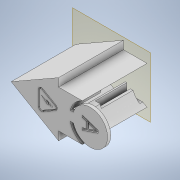
# Autodesk Inventor part: Wire_Closing_3
Saved by Autodesk Inventor 2022.3 (Build 263350000, 350)
## iProperties
Created: 2023-05-07
Part Number: Wire_Closing_3
Material: Generic
Document SubType Name: Modeling
Designer: Manuel Hueso Béjar
Density: 1 g/cm^3
Appearance: Default
Author: Manuel Hueso Béjar
Autodesk Inventor part; units mm, degrees
ref_plane "YZ Plane" through (0, 0, 0) normal (1, 0, 0) x (0, 1, 0)
ref_plane "XZ Plane" through (0, 0, 0) normal (0, 1, 0) x (-1, 0, 0)
ref_plane "XY Plane" through (0, 0, 0) normal (0, 0, 1) x (1, 0, 0)
ref_plane "Work Plane1" through (0, 0, 0) normal (0, 0, 1) x (1, 0, 0)
sketch "Sketch1" plane through (0, 0, 0) normal (0, 0, 1) x (1, 0, 0)
  line L0 (7.4997, 17.3208) -> (7.4997, 12.145) projected
  line L1 (-22.5003, 0.1452) -> (7.4997, 17.3208) projected
  line L2 (7.4997, -17.3208) -> (-22.5003, 0.1452) projected
  line L3 (7.4997, -11.855) -> (7.4997, -17.3208) projected
  line L4 (22.5003, -11.855) -> (7.4997, -11.855) projected
  arc A0 (19.8352, -10.355) -> (22.5003, -11.855) centre (27.4997, 0.1452) ccw projected
  line L5 (5.9997, -10.355) -> (19.8352, -10.355) projected
  line L6 (5.9997, -14.7118) -> (5.9997, -10.355) projected
  line L7 (-19.5003, 0.1343) -> (5.9997, -14.7118) projected
  line L8 (5.9997, 14.7336) -> (-19.5003, 0.1343) projected
  line L9 (5.9997, 10.645) -> (5.9997, 14.7336) projected
  line L10 (19.8345, 10.645) -> (5.9997, 10.645) projected
  arc A1 (22.4991, 12.145) -> (19.8345, 10.645) centre (27.4997, 0.1452) ccw projected
  line L11 (7.4997, 12.145) -> (22.4991, 12.145) projected
  point P0 (0, 0)
extrude "Extrusion1" add sketch "Sketch1" along normal blind 41
sketch "Sketch2" plane through (0, 0, 41) normal (0, 0, 1) x (1, 0, 0)
  line L0 (-22.5003, 0.1452) -> (7.4997, -17.3208) projected
  line L1 (7.4997, -17.3208) -> (7.4997, -11.855) projected
  line L2 (7.4997, -11.855) -> (22.5003, -11.855) projected
  arc A0 (19.8352, -10.355) -> (22.5003, -11.855) centre (27.4997, 0.1452) ccw projected
  line L3 (19.8352, -10.355) -> (5.9997, -10.355) projected
  line L4 (5.9997, -10.355) -> (5.9997, -14.7118) projected
  line L5 (5.9997, -14.7118) -> (-19.5003, 0.1343) projected
  line L6 (-19.5003, 0.1343) -> (5.9997, 14.7336) projected
  line L7 (5.9997, 14.7336) -> (5.9997, 10.645) projected
  line L8 (5.9997, 10.645) -> (19.8345, 10.645) projected
  arc A1 (22.4991, 12.145) -> (19.8345, 10.645) centre (27.4997, 0.1452) ccw projected
  line L9 (22.4991, 12.145) -> (7.4997, 12.145) projected
  line L10 (7.4997, 12.145) -> (7.4997, 17.3208) projected
  line L11 (7.4997, 17.3208) -> (-22.5003, 0.1452) projected
  arc A2 (22.4991, 12.145) -> (19.8345, 10.645) centre (27.4997, 0.1452) ccw projected
  arc A3 (22.4991, 12.145) -> (22.5003, -11.855) centre (27.4997, 0.1452) ccw
  arc A4 (16.9167, -2.8548) -> (16.9167, 3.1452) centre (27.4997, 0.1452) ccw projected
  line L12 (16.9167, -2.8548) -> (14.8506, -2.8548) projected
  arc A5 (14.8506, -2.8548) -> (14.8506, 3.1452) centre (27.4997, 0.1452) ccw projected
  line L13 (14.8506, 3.1452) -> (16.9167, 3.1452) projected
  point P0 (0, 0)
  constraints: 3 point on circle, 2 end point, 1 centre point, 1 coincident
extrude "Extrusion2" add sketch "Sketch2" against normal blind 2 contours L3 L4 L5 L6 L7 L8 A3 | A3 L13 A4 L12
sketch "Sketch3" plane through (0, 0, 39) normal (0, 0, -1) x (-1, 0, 0)
  line L0 (-15.4997, 5.1452) -> (-13.8506, 5.1452) projected
  line L1 (-13.8506, 5.1452) -> (-11.8506, 7.1452) projected
  line L2 (-11.8506, 7.1452) -> (-11.8506, 3.1452) projected
  line L3 (-11.8506, 3.1452) -> (-14.8506, 3.1452) projected
  arc A0 (-14.8506, 3.1452) -> (-15.4997, 5.1452) centre (-27.4997, 0.1452) ccw projected
  arc A1 (-15.4997, -4.8548) -> (-14.8506, -2.8548) centre (-27.4997, 0.1452) ccw projected
  line L4 (-14.8506, -2.8548) -> (-11.8506, -2.8548) projected
  line L5 (-11.8506, -2.8548) -> (-11.8506, -6.8548) projected
  line L6 (-11.8506, -6.8548) -> (-13.8506, -4.8548) projected
  line L7 (-13.8506, -4.8548) -> (-15.4997, -4.8548) projected
  line L8 (-5.9997, 14.7336) -> (19.5003, 0.1343) projected
  line L9 (-5.9997, 10.645) -> (-5.9997, 14.7336) projected
  line L10 (-19.8345, 10.645) -> (-5.9997, 10.645) projected
  arc A2 (-14.8506, 3.1452) -> (-19.8345, 10.645) centre (-27.4997, 0.1452) ccw projected
  line L11 (-14.8506, 3.1452) -> (-16.9167, 3.1452) projected
  arc A3 (-16.9167, 3.1452) -> (-16.9167, -2.8548) centre (-27.4997, 0.1452) ccw projected
  line L12 (-16.9167, -2.8548) -> (-14.8506, -2.8548) projected
  arc A4 (-19.8352, -10.355) -> (-14.8506, -2.8548) centre (-27.4997, 0.1452) ccw projected
  line L13 (-5.9997, -10.355) -> (-19.8352, -10.355) projected
  line L14 (-5.9997, -14.7118) -> (-5.9997, -10.355) projected
  line L15 (19.5003, 0.1343) -> (-5.9997, -14.7118) projected
  line L16 (-13.9334, -5.0548) -> (-11.6506, -7.3376)
  line L17 (-11.6506, -7.3376) -> (-11.6506, -2.6548)
  line L18 (-11.6506, -2.6548) -> (-15.0097, -2.6548)
  arc A5 (-15.8035, -5.0548) -> (-15.0097, -2.6548) centre (-27.4997, 0.1452) ccw
  line L19 (-15.8035, -5.0548) -> (-13.9334, -5.0548)
  line L20 (-11.6506, 2.9452) -> (-11.6506, 7.6281)
  line L21 (-11.6506, 7.6281) -> (-13.9334, 5.3452)
  line L22 (-13.9334, 5.3452) -> (-15.8035, 5.3452)
  arc A6 (-15.0097, 2.9452) -> (-15.8035, 5.3452) centre (-27.4997, 0.1452) ccw
  line L23 (-15.0097, 2.9452) -> (-11.6506, 2.9452)
  line L24 (-11.8506, -2.8548) -> (-11.6506, -2.8548)
  line L25 (-11.8506, 3.1452) -> (-11.6506, 3.1452)
  line L26 (-10.6506, -9.7518) -> (-14.3476, -6.0548)
  line L27 (-14.3476, -6.0548) -> (-17.4598, -6.0548)
  arc A7 (-17.4598, -6.0548) -> (-15.8378, -1.6548) centre (-27.4997, 0.1452) ccw
  line L28 (-15.8378, -1.6548) -> (-10.6506, -1.6548)
  line L29 (-10.6506, -1.6548) -> (-10.6506, -9.7518)
  line L30 (-14.3476, 6.3452) -> (-10.6506, 10.0423)
  line L31 (-10.6506, 10.0423) -> (-10.6506, 1.9452)
  line L32 (-10.6506, 1.9452) -> (-15.8378, 1.9452)
  arc A8 (-15.8378, 1.9452) -> (-17.4598, 6.3452) centre (-27.4997, 0.1452) ccw
  line L33 (-17.4598, 6.3452) -> (-14.3476, 6.3452)
  line L34 (-11.6506, -2.8548) -> (-10.6506, -2.8548)
  line L35 (-11.6506, 3.1452) -> (-10.6506, 3.1452)
  point P0 (0, 0)
  point P1 (-16.0734, 6.3452)
  point P2 (-15.585, 5.3452)
  point P3 (-15.585, -5.0548)
  point P4 (-16.0734, -6.0548)
  dimension "d4" = 0.2
  dimension "d5" = 0.2
  dimension "d6" = 1
  dimension "d7" = 1
  constraints: 40 end point, 8 point on circle, 4 centre point, 4 perpendicular, 4 point on line, 16 other
  measures "d4" distance between parallel lines of L6 L16
  measures "d5" distance between parallel lines of L2 L20
  measures "d6" distance between parallel lines of L16 L26
  measures "d7" distance between parallel lines of L21 L30
extrude "Extrusion3" add sketch "Sketch3" along normal blind 37 contours A2 L33 L30 L31 L35 L20 L21 L22 | A4 L19 L16 L17 L34 L29 L26 L27
sketch "Sketch4" plane through (0, 0, 39) normal (0, 0, -1) x (-1, 0, 0)
  line L0 (-16.0734, 6.3452) -> (-14.3476, 6.3452) projected
  line L1 (-14.3476, 6.3452) -> (-10.6506, 10.0423) projected
  line L2 (-10.6506, 10.0423) -> (-10.6506, 3.1452) projected
  line L3 (-10.6506, 3.1452) -> (-11.6506, 3.1452) projected
  line L4 (-11.6506, 3.1452) -> (-11.6506, 7.6281) projected
  line L5 (-11.6506, 7.6281) -> (-13.9334, 5.3452) projected
  line L6 (-13.9334, 5.3452) -> (-15.585, 5.3452) projected
  arc A0 (-14.8506, 3.1452) -> (-15.585, 5.3452) centre (-27.4997, 0.1452) ccw projected
  line L7 (-14.8506, 3.1452) -> (-16.9167, 3.1452) projected
  arc A1 (-16.9167, 3.1452) -> (-16.9167, -2.8548) centre (-27.4997, 0.1452) ccw projected
  line L8 (-16.9167, -2.8548) -> (-14.8506, -2.8548) projected
  arc A2 (-15.585, -5.0548) -> (-14.8506, -2.8548) centre (-27.4997, 0.1452) ccw projected
  line L9 (-15.585, -5.0548) -> (-13.9334, -5.0548) projected
  line L10 (-13.9334, -5.0548) -> (-11.6506, -7.3376) projected
  line L11 (-11.6506, -7.3376) -> (-11.6506, -2.8548) projected
  line L12 (-11.6506, -2.8548) -> (-10.6506, -2.8548) projected
  line L13 (-10.6506, -2.8548) -> (-10.6506, -9.7518) projected
  line L14 (-10.6506, -9.7518) -> (-14.3476, -6.0548) projected
  line L15 (-14.3476, -6.0548) -> (-16.0734, -6.0548) projected
  arc A3 (-19.8352, -10.355) -> (-16.0734, -6.0548) centre (-27.4997, 0.1452) ccw projected
  line L16 (-5.9997, -10.355) -> (-19.8352, -10.355) projected
  line L17 (-5.9997, -14.7118) -> (-5.9997, -10.355) projected
  line L18 (19.5003, 0.1343) -> (-5.9997, -14.7118) projected
  line L19 (-5.9997, 14.7336) -> (19.5003, 0.1343) projected
  line L20 (-5.9997, 10.645) -> (-5.9997, 14.7336) projected
  line L21 (-19.8345, 10.645) -> (-5.9997, 10.645) projected
  arc A4 (-16.0734, 6.3452) -> (-19.8345, 10.645) centre (-27.4997, 0.1452) ccw projected
  line L22 (-14.8506, 3.1452) -> (-16.9167, 3.1452) projected
  line L23 (-14.8506, 3.1452) -> (-11.6506, 3.1452)
  arc A5 (-22.5003, -11.855) -> (-14.8506, -2.8548) centre (-27.4997, 0.1452) ccw projected
  line L24 (-11.6506, -7.3376) -> (-11.6506, -2.8548) projected
  line L25 (-14.8506, -2.8548) -> (-11.6506, -2.8548)
  point P0 (0, 0)
  constraints: 4 end point, 1 collinear, 1 horizontal
extrude "Extrusion4" add sketch "Sketch4" along normal blind 17 contours L23 A0 L6 L5 L4 | L25 L11 L10 L9 A2
sketch "Sketch5" plane through (0, 0, 39) normal (0, 0, -1) x (-1, 0, 0)
  line L0 (-14.8506, -2.8548) -> (-10.6506, -2.8548) projected
  line L1 (-10.6506, -2.8548) -> (-10.6506, -9.7518) projected
  line L2 (-10.6506, -9.7518) -> (-14.3476, -6.0548) projected
  line L3 (-14.3476, -6.0548) -> (-16.0734, -6.0548) projected
  arc A0 (-19.8352, -10.355) -> (-16.0734, -6.0548) centre (-27.4997, 0.1452) ccw projected
  line L4 (-5.9997, -10.355) -> (-19.8352, -10.355) projected
  line L5 (-5.9997, -14.7118) -> (-5.9997, -10.355) projected
  line L6 (19.5003, 0.1343) -> (-5.9997, -14.7118) projected
  line L7 (-5.9997, 14.7336) -> (19.5003, 0.1343) projected
  line L8 (-5.9997, 10.645) -> (-5.9997, 14.7336) projected
  line L9 (-19.8345, 10.645) -> (-5.9997, 10.645) projected
  arc A1 (-16.0734, 6.3452) -> (-19.8345, 10.645) centre (-27.4997, 0.1452) ccw projected
  line L10 (-16.0734, 6.3452) -> (-14.3476, 6.3452) projected
  line L11 (-14.3476, 6.3452) -> (-10.6506, 10.0423) projected
  line L12 (-10.6506, 10.0423) -> (-10.6506, 3.1452) projected
  line L13 (-10.6506, 3.1452) -> (-14.8506, 3.1452) projected
  line L14 (-14.8506, 3.1452) -> (-16.9167, 3.1452) projected
  arc A2 (-16.9167, 3.1452) -> (-16.9167, -2.8548) centre (-27.4997, 0.1452) ccw projected
  line L15 (-16.9167, -2.8548) -> (-14.8506, -2.8548) projected
  line L16 (-10.6506, 10.0423) -> (-14.3476, 6.3452) projected
  line L17 (-10.6506, 10.0423) -> (-10.6506, 10.645)
  line L18 (-19.8345, 10.645) -> (-5.9997, 10.645) projected
  line L19 (-10.6506, -9.7518) -> (-14.3476, -6.0548) projected
  line L20 (-10.6506, -9.7518) -> (-10.6506, -10.355)
  line L21 (-5.9997, -10.355) -> (-19.8352, -10.355) projected
  point P0 (0, 0)
  constraints: 4 end point, 2 point on line, 1 perpendicular, 1 vertical
extrude "Extrusion5" add sketch "Sketch5" along normal up to surface (37 mm away) contours L20 L4 A0 L3 L2 | L11 L10 A1 L9 L17
sketch "Sketch6" plane through (0, 0, 41) normal (0, 0, 1) x (1, 0, 0)
  line L0 (3.39, -1.0702) -> (-3.39, -1.0702)
  line L1 (-3.39, -1.0702) -> (-3.39, 2.3198)
  line L2 (3.39, -1.0702) -> (3.39, 0.6248)
  line L3 (0, -1.0702) -> (1.695, -1.0702)
  line L4 (1.695, -1.0702) -> (0, -1.0702)
  line L5 (0.8475, -1.0702) -> (0, -1.0702)
  line L6 (-3.39, 2.3198) -> (0, 0.6248) construction
  line L7 (0.8475, 0.201) -> (3.39, -1.0702) construction
  line L8 (3.39, -0.2227) -> (0, 1.4723)
  line L9 (0, 1.4723) -> (0, 0.6248)
  line L10 (0, 0.6248) -> (-3.39, 2.3198)
  line L11 (5.4636, -0.8745) -> (-2.8833, -5.6936)
  line L12 (-2.8833, 5.6766) -> (5.4636, 0.8575)
  arc A0 (5.4636, -0.8745) -> (5.4636, 0.8575) centre (4.9636, -0.0085) ccw
  arc A1 (-2.8833, 5.6766) -> (-4.3833, 4.8105) centre (-3.3833, 4.8105) ccw
  arc A2 (-4.3833, -4.8276) -> (-2.8833, -5.6936) centre (-3.3833, -4.8276) ccw
  line L13 (5.8386, 1.507) -> (-2.5083, 6.3261)
  arc A3 (-2.5083, 6.3261) -> (-5.1333, 4.8105) centre (-3.3833, 4.8105) ccw
  line L14 (-5.1333, 4.8105) -> (-5.1333, -4.8276)
  arc A4 (-5.1333, -4.8276) -> (-2.5083, -6.3431) centre (-3.3833, -4.8276) ccw
  line L15 (-2.5083, -6.3431) -> (5.8386, -1.524)
  arc A5 (5.8386, -1.524) -> (5.8386, 1.507) centre (4.9636, -0.0085) ccw
  line L16 (-3.39, 2.3198) -> (0.8475, -1.0702)
  line L17 (0.8475, -1.0702) -> (0.8475, 0.201)
  line L18 (0.8475, 0.201) -> (3.39, -1.0702)
  line L19 (3.39, -0.2227) -> (3.39, -1.0702)
  line L20 (-4.3833, 4.8105) -> (-4.3833, -4.8276)
  point P0 (7.5646, 0.6248)
  point P1 (-3.7823, -5.9263)
  point P2 (-3.7823, 7.1759)
  dimension "d28" = 1
  dimension "d29" = 1
  dimension "d30" = 0.75
  constraints: 42 end point, 12 point on circle, 6 centre point, 4 tangent, 3 collinear, 3 midpoint, 2 horizontal, 2 vertical, 1 coincident, 1 equal radius, 1 perpendicular, 7 other
  measures "d28" radius of A0
  measures "d29" radius of A1
  measures "d30" distance between parallel lines of L12 L13
sketch "Sketch7" plane through (0, 0, 41) normal (0, 0, 1) x (1, 0, 0)
  line L0 (38.4997, 11.1452) -> (38.4997, -10.8548) construction
  line L1 (38.4997, -10.8548) -> (16.4997, -10.8548) construction
  line L2 (16.4997, -10.8548) -> (16.4997, 11.1452) construction
  line L3 (16.4997, 11.1452) -> (38.4997, 11.1452) construction
  line L4 (38.4997, 11.1452) -> (16.4997, 11.1452)
  line L5 (16.4997, 11.1452) -> (16.4997, -10.8548)
  line L6 (16.4997, -10.8548) -> (38.4997, -10.8548)
  line L7 (38.4997, -10.8548) -> (38.4997, 11.1452)
  arc A0 (16.9167, -2.8548) -> (16.9167, 3.1452) centre (27.4997, 0.1452) ccw projected
  line L8 (38.4997, 11.1452) -> (16.4997, -10.8548) construction
  line L9 (16.4997, 11.1452) -> (38.4997, -10.8548) construction
  line L10 (22.4997, 4.3997) -> (32.4997, 1.0285)
  line L11 (32.4997, 1.0285) -> (32.4997, -0.6084)
  line L12 (32.4997, -0.6084) -> (22.4997, -3.9796)
  line L13 (22.4997, -3.9796) -> (22.4997, -2.5776)
  line L14 (22.4997, -2.5776) -> (25.2955, -1.67)
  line L15 (25.2955, -1.67) -> (25.2955, 2.1469)
  line L16 (25.2955, 2.1469) -> (22.4997, 3.0545)
  line L17 (22.4997, 3.0545) -> (22.4997, 4.3997)
  line L18 (26.43, -1.3053) -> (31.1383, 0.2425)
  line L19 (31.1383, 0.2425) -> (26.43, 1.7822)
  line L20 (26.43, 1.7822) -> (26.43, -1.3053)
  point P0 (0, 0)
  dimension "d19" = 22
  dimension "d20" = 22
  dimension "d21" = 22
  dimension "d22" = 22
  dimension "d23" = 0
  dimension "d24" = 0
  constraints: 12 end point, 2 midpoint, 2 parallel, 1 horizontal, 1 perpendicular, 2 other
  measures "d19" distance of L0.start L0.end
  measures "d20" distance of L2.end L0.start
  measures "d21" distance of L6.end L5.end
  measures "d22" distance of L5.end L4.end
  measures "d23" distance between parallel lines of L7 L0
  measures "d24" distance between parallel lines of L3 L4
emboss "Emboss2" sketch "Sketch7" operation cut depth 1 direction (0, 0, -1) contours L10 L11 L12 L13 L14 L15 L16 L17
emboss "Emboss3" sketch "Sketch6" operation cut depth 1 direction (0, 0, -1) contours L18 L17 L16 L10 L9 L8 L2 | A5 L15 A4 L14 A3 L13
body "Solid1"
